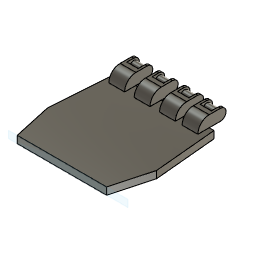
baseplate with holes (Autodesk Fusion 360 design; units mm, degrees)
Autodesk Fusion 360 part; units mm, degrees
sketch "Sketch1" plane through (0, 0, 0) normal (0, 0, 1) x (1, 0, 0)
  line L0 (0, 0) -> (76, 0)
  line L1 (76, 0) -> (76, 76)
  line L2 (76, 76) -> (0, 76)
  line L3 (0, 76) -> (0, 0)
  dimension "d1" = 76
  dimension "d2" = 76
  constraint horizontal L0
  constraint vertical L1
  constraint horizontal L2
  constraint vertical L3
  constraint coincident L0.start L3.end
  measures "d1" distance of L0.start L0.end
  measures "d2" distance of L0.start L2.end
extrude "Extrude1" add sketch "Sketch1" along normal blind 6.35
sketch "Sketch2" plane through (0, 0, 6.35) normal (0, 0, 1) x (-1, 0, 0)
  line L0 (0, -76) -> (0, 0)
  line L1 (0, 0) -> (-76, 0)
  line L2 (-76, 0) -> (-76, -76)
  line L3 (-76, -76) -> (0, -76)
  line L4 (-52, -66) -> (-38, -66)
  line L5 (-38, -66) -> (-38, -91)
  line L6 (-38, -91) -> (-52, -91)
  line L7 (-52, -91) -> (-52, -66)
  line L8 (-34.5, -66) -> (-20.5, -66)
  line L9 (-34.5, -91) -> (-34.5, -66)
  line L10 (-20.5, -66) -> (-20.5, -91)
  line L11 (-20.5, -91) -> (-34.5, -91)
  line L12 (-17, -66) -> (-3, -66)
  line L13 (-17, -91) -> (-17, -66)
  line L14 (-3, -66) -> (-3, -91)
  line L15 (-3, -91) -> (-17, -91)
  line L16 (-72, -66) -> (-58, -66)
  line L17 (-72, -91) -> (-72, -66)
  line L18 (-58, -66) -> (-58, -91)
  line L19 (-58, -91) -> (-72, -91)
  dimension "d5" = 14
  dimension "d6" = 25
  dimension "d7" = 24
  dimension "d8" = 10
  dimension "d89" = 35
  dimension "d90" = 0
  dimension "d93" = -20
  dimension "d94" = 0
  constraint horizontal L4
  constraint vertical L5
  constraint horizontal L6
  constraint vertical L7
  measures "d5" distance of L4.start L4.end
  measures "d6" distance of L4.start L6.end
  measures "d7" distance of L2 L7
  measures "d8" distance of L3 L4
extrude "Extrude2" add sketch "Sketch2" along normal blind 10 contours L3 L5 L6 L7 | L3 L4 L5 L7
fillet "Fillet1" radius 10 1 edges at (45, 66, 16.35)
fillet "Fillet2" radius 5 2 edges at (45, 91, 16.35) (45, 91, 6.35)
sketch "Sketch3" plane through (0, 0, 16.35) normal (0, 0, 1) x (-1, 0, 0)
  line L0 (-52, -86) -> (-38, -86)
  line L1 (-38, -86) -> (-38, -76)
  line L2 (-38, -76) -> (-52, -76)
  line L3 (-52, -76) -> (-52, -86)
  line L4 (-50, -80) -> (-40, -80)
  line L5 (-40, -80) -> (-40, -95)
  line L6 (-40, -95) -> (-50, -95)
  line L7 (-50, -95) -> (-50, -80)
  constraint horizontal L4
  constraint vertical L5
  constraint horizontal L6
  constraint vertical L7
extrude "Extrude3" cut sketch "Sketch3" against normal blind 20 contours L0 L4 L5 L7 | L0 L5 L6 L7
sketch "Sketch4" plane through (40, 0, 0) normal (1, 0, 0) x (0, 1, 0)
  line L0 (80, 6.35) -> (86, 6.35)
  arc A0 (86, 6.35) -> (86, 16.35) centre (86, 11.35) ccw
  line L1 (86, 16.35) -> (80, 16.35)
  line L2 (80, 16.35) -> (80, 6.35)
  circle A1 centre (86, 11.35) radius 3.25
  dimension "d17" = 6.5
  constraint concentric A0 A1
  measures "d17" diameter of A1
extrude "Extrude4" add sketch "Sketch4" along normal blind 10 contours A1
extrude "Extrude5" add 1 faces at (76, 25.3333, 2.1167) along direction (1, 0, 0) blind 5
extrude "Extrude6" add 1 faces at (0, 50.6667, 2.1167) along direction (-1, 0, 0) blind 5
extrude "Extrude7" add 1 faces at (23.6667, 0, 2.1167) along direction (0, -1, 0) blind 5
sketch "Sketch5" plane through (0, 0, 6.35) normal (0, 0, 1) x (-1, 0, 0)
  line L0 (-38, -66) -> (-38, -76)
  line L1 (-38, -76) -> (5, -76)
  line L2 (5, -76) -> (5, 5)
  line L3 (5, 5) -> (-81, 5)
  line L4 (-81, 5) -> (-81, -76)
  line L5 (-81, -76) -> (-52, -76)
  line L6 (-52, -76) -> (-52, -66)
  line L7 (-52, -66) -> (-38, -66)
  line L8 (-81, -76) -> (-76.6575, -76)
  line L9 (-76.6575, -76) -> (-76.6575, -71)
  line L10 (-76.6575, -71) -> (-81, -71)
  line L11 (-81, -71) -> (-81, -76)
  line L12 (5, -76) -> (0, -76)
  line L13 (0, -76) -> (0, -71)
  line L14 (0, -71) -> (5, -71)
  line L15 (5, -71) -> (5, -76)
  line L16 (5, 5) -> (0, 5)
  line L17 (0, 5) -> (0, 0)
  line L18 (0, 0) -> (5, 0)
  line L19 (5, 0) -> (5, 5)
  line L20 (-81, 5) -> (-76, 5)
  line L21 (-76, 5) -> (-76, 0)
  line L22 (-76, 0) -> (-81, 0)
  line L23 (-81, 0) -> (-81, 5)
  dimension "d26" = 5
  dimension "d27" = 5
  dimension "d28" = 5
  dimension "d29" = 5
  dimension "d30" = 5
  dimension "d31" = 5
  dimension "d32" = 5
  constraint horizontal L8
  constraint vertical L9
  constraint horizontal L10
  constraint vertical L11
  constraint coincident L4.end L5.start
  constraint horizontal L12
  constraint vertical L13
  constraint horizontal L14
  constraint vertical L15
  constraint coincident L1.end L2.start
  constraint horizontal L16
  constraint vertical L17
  constraint horizontal L18
  constraint vertical L19
  constraint coincident L2.end L3.start
  constraint horizontal L20
  constraint vertical L21
  constraint horizontal L22
  constraint vertical L23
  constraint coincident L3.end L4.start
  measures "d26" distance of L4.end L10.end
  measures "d27" distance of L1.end L12.end
  measures "d28" distance of L1.end L14.end
  measures "d29" distance of L2.end L16.end
  measures "d30" distance of L2.end L18.end
  measures "d31" distance of L3.end L20.end
  measures "d32" distance of L3.end L22.end
sketch "Sketch7" plane through (0, 0, 6.35) normal (0, 0, 1) x (-1, 0, 0)
  line L0 (5, 5) -> (-81, 5)
  line L1 (-81, 5) -> (-81, -76)
  line L2 (-38, -76) -> (5, -76)
  line L3 (-52, -76) -> (-52, -66)
  line L4 (-52, -66) -> (-38, -66)
  line L5 (-38, -66) -> (-38, -76)
  line L6 (5, -76) -> (5, 5)
  circle A0 centre (-38, -24.9192) radius 1
  circle A1 centre (-64, -24.9192) radius 1
  line L7 (-81, -76) -> (-52, -76)
  dimension "d35" = 2
  dimension "d36" = 2
  dimension "d39" = 26
  measures "d35" diameter of A1
  measures "d36" diameter of A0
  measures "d39" distance of A0.centre A1.centre
extrude "Extrude11" add 1 faces at (81, 22, 2.1167) along direction (1, 0, 0) blind 10
extrude "Extrude12" add 1 faces at (59, -5, 4.2333) along direction (0, -1, 0) blind 10
extrude "Extrude13" add 1 faces at (-5, 45.6667, 2.1167) along direction (-1, 0, 0) blind 10
sketch "Sketch10" plane through (0, -15, 0) normal (0, -1, 0) x (1, 0, 0)
  line L0 (-15, 0) -> (91, 0)
  line L1 (91, 0) -> (91, 6.35)
  line L2 (91, 6.35) -> (-15, 6.35)
  line L3 (-15, 6.35) -> (-15, 0)
sketch "Sketch11" plane through (0, 0, 0) normal (0, 0, 1) x (1, 0, 0)
  line L0 (91, 76) -> (96, 76)
  line L1 (96, 76) -> (96, 71)
  line L2 (96, 71) -> (91, 71)
  line L3 (91, 71) -> (91, 76)
  line L4 (-15, 76) -> (-20, 76)
  line L5 (-20, 76) -> (-20, 71)
  line L6 (-20, 71) -> (-15, 71)
  line L7 (-15, 71) -> (-15, 76)
  line L8 (91, -15) -> (86, -15)
  line L9 (86, -15) -> (86, -20)
  line L10 (86, -20) -> (91, -20)
  line L11 (91, -20) -> (91, -15)
  line L12 (-15, -15) -> (-10, -15)
  line L13 (-10, -15) -> (-10, -20)
  line L14 (-10, -20) -> (-15, -20)
  line L15 (-15, -20) -> (-15, -15)
  dimension "d70" = 5
  dimension "d71" = 5
  dimension "d72" = 5
  dimension "d73" = 5
  dimension "d74" = 5
  dimension "d75" = 5
  dimension "d76" = 5
  dimension "d77" = 5
  constraint horizontal L0
  constraint vertical L1
  constraint horizontal L2
  constraint vertical L3
  constraint horizontal L4
  constraint vertical L5
  constraint horizontal L6
  constraint vertical L7
  constraint horizontal L8
  constraint vertical L9
  constraint horizontal L10
  constraint vertical L11
  constraint horizontal L12
  constraint vertical L13
  constraint horizontal L14
  constraint vertical L15
  measures "d70" distance of L0.start L0.end
  measures "d71" distance of L0.start L2.end
  measures "d72" distance of L4.start L4.end
  measures "d73" distance of L4.start L6.end
  measures "d74" distance of L8.start L8.end
  measures "d75" distance of L8.start L10.end
  measures "d76" distance of L12.start L12.end
  measures "d77" distance of L12.start L14.end
sketch "Sketch12" plane through (0, 0, 0) normal (0, 0, 1) x (1, 0, 0)
  arc A0 (91, -20) -> (96, 71) centre (-640.4348, 65.8261) ccw
  arc A1 (-20, 71) -> (-15, -20) centre (801.5, 70.5) ccw
  arc A2 (-10, -20) -> (86, -20) centre (38, 315.1878) ccw
  line L0 (-20, 71) -> (-15, 71)
  line L1 (-15, 71) -> (-15, -20)
  line L2 (-10, -20) -> (-10, -14.8)
  line L3 (-10, -14.8) -> (86, -14)
  line L4 (86, -14) -> (86, -20)
  line L5 (96, 71) -> (90, 71)
  line L6 (90, 71) -> (90, -20)
  line L7 (90, -20) -> (91, -20)
  point P0 (-9.9984, -14.9986)
  constraint horizontal L0
  constraint vertical L2
  constraint parallel L2 L4
  constraint perpendicular L4 L5
  constraint perpendicular L5 L6
  constraint perpendicular L6 L7
pattern_linear "R-Pattern1" count 3 spacing 22.5 along (-1, 0, 0) of "Extrude2", "Fillet1", "Fillet2", "Extrude3", "Extrude4"
pattern_linear "R-Pattern2" count 2 spacing 20 along (1, 0, 0) of "Extrude2", "Fillet1", "Fillet2", "Extrude3", "Extrude4"
sketch "Sketch14" plane through (0, 0, 6.35) normal (0, 0, 1) x (-1, 0, 0)
  line L0 (-58, -66) -> (-58, -76)
  line L1 (-58, -76) -> (-52, -76)
  line L2 (-52, -76) -> (-52, -66)
  line L3 (-52, -66) -> (-38, -66)
  line L4 (-38, -66) -> (-38, -76)
  line L5 (-38, -76) -> (-29.5, -76)
  line L6 (-29.5, -76) -> (-29.5, -66)
  line L7 (-29.5, -66) -> (-15.5, -66)
  line L8 (-15.5, -66) -> (-15.5, -76)
  line L9 (-15.5, -76) -> (-7, -76)
  line L10 (-7, -76) -> (-7, -66)
  line L11 (-7, -66) -> (7, -66)
  line L12 (7, -66) -> (7, -76)
  line L13 (7, -76) -> (15, -76)
  line L14 (15, -76) -> (15, 15)
  line L15 (15, 15) -> (-91, 15)
  line L16 (-91, 15) -> (-91, -76)
  line L17 (-91, -76) -> (-72, -76)
  line L18 (-72, -76) -> (-72, -66)
  line L19 (-72, -66) -> (-58, -66)
  line L20 (-76.2804, -76) -> (-81.5, -19.824)
  line L21 (-81.5, -19.824) -> (-72, 15)
  line L22 (-72, 15) -> (7.2884, 15)
  line L23 (11, -76) -> (15, -19.824)
  line L24 (15, -19.824) -> (7.2884, 15)
  dimension "d105" = 56.176
  dimension "d106" = 56.176
  dimension "d107" = 102.486
  dimension "d108" = 105.259
  dimension "d109" = 87.2804
  dimension "d110" = 159.433
  constraint coincident L17 L20.start
  constraint coincident L15 L21.end
  constraint coincident L15 L22.end
  constraint midpoint L13 L23.start
  constraint coincident L14 L23.end
  measures "d105" vertical distance of L20.start L20.end
  measures "d106" vertical distance of L23.start L23.end
  measures "d107" angle of L22 L24
  measures "d108" angle of L21 L22
  measures "d109" distance of L20.start L23.start
  measures "d110" angle of L20 L21
extrude "Extrude17" cut sketch "Sketch14" against normal blind 10 contours L15 L16 L17 L20 L21 | L14 L15 L24 | L13 L14 L23
sketch "Sketch15" plane through (0, 0, 0) normal (0, 0, -1) x (1, 0, 0)
  line L0 (-15, -19.824) -> (-11, -76)
  line L1 (-11, -76) -> (76.2804, -76)
  line L2 (76.2804, -76) -> (81.5, -19.824)
  line L3 (81.5, -19.824) -> (72, 15)
  line L4 (72, 15) -> (-7.2884, 15)
  line L5 (-7.2884, 15) -> (-15, -19.824)
  line L6 (73.0232, -74) -> (57.0232, -74)
  line L7 (57.0232, -74) -> (57.0232, -25.5)
  line L8 (57.0232, -25.5) -> (73.0232, -25.5)
  line L9 (73.0232, -25.5) -> (73.0232, -74)
  line L10 (52.9695, -74) -> (36.9695, -74)
  line L11 (36.9695, -74) -> (36.9695, -25.5)
  line L12 (36.9695, -25.5) -> (52.9695, -25.5)
  line L13 (52.9695, -25.5) -> (52.9695, -74)
  line L14 (30.4888, -74) -> (14.4888, -74)
  line L15 (14.4888, -74) -> (14.4888, -25.5)
  line L16 (14.4888, -25.5) -> (30.4888, -25.5)
  line L17 (30.4888, -25.5) -> (30.4888, -74)
  line L18 (8.0069, -74) -> (-7.9931, -74)
  line L19 (-7.9931, -74) -> (-7.9931, -25.5)
  line L20 (-7.9931, -25.5) -> (8.0069, -25.5)
  line L21 (8.0069, -25.5) -> (8.0069, -74)
  dimension "d113" = 16
  dimension "d114" = 16
  dimension "d115" = 16
  dimension "d116" = 16
  dimension "d117" = 48.5
  dimension "d118" = 48.5
  dimension "d119" = 48.5
  dimension "d120" = 48.5
  dimension "d121" = 2
  dimension "d122" = 2
  dimension "d123" = 2
  dimension "d124" = 2
  dimension "d125" = 4.0537
  dimension "d126" = 90
  dimension "d127" = 6.4807
  dimension "d128" = 6.4819
  dimension "d129" = 3.2572
  constraint parallel L1 L6
  constraint perpendicular L6 L7
  constraint perpendicular L7 L8
  constraint perpendicular L6 L9
  constraint perpendicular L9 L10
  constraint perpendicular L10 L11
  constraint perpendicular L11 L12
  constraint perpendicular L10 L13
  constraint perpendicular L11 L14
  constraint perpendicular L14 L15
  constraint perpendicular L15 L16
  constraint perpendicular L15 L18
  constraint perpendicular L18 L19
  constraint perpendicular L19 L20
  constraint perpendicular L18 L21
  measures "d113" distance of L6.start L6.end
  measures "d114" distance of L10.start L10.end
  measures "d115" distance of L14.start L14.end
  measures "d116" distance of L18.start L18.end
  measures "d117" distance of L18.end L19.end
  measures "d118" distance of L14.end L15.end
  measures "d119" distance of L10.end L11.end
  measures "d120" distance of L6.start L8.end
  measures "d121" distance of L1 L6
  measures "d122" distance of L1 L10
  measures "d123" distance of L1 L18
  measures "d124" distance of L1 L14
  measures "d125" distance of L7 L13
  measures "d126" angle of L16 L17
  measures "d127" distance of L11 L17
  measures "d128" distance of L15 L21
  measures "d129" horizontal distance of L1.end L6.start
extrude "Extrude18" cut sketch "Sketch15" against normal blind 5 contours L6 L7 L8 L9 | L10 L11 L12 L13 | L14 L15 L16 L17 | L18 L19 L20 L21
sketch "Sketch16" plane through (0, 0, 0) normal (0, 0, -1) x (1, 0, 0)
  line L0 (36.9695, -74) -> (36.9695, -25.5)
  line L1 (36.9695, -25.5) -> (52.9695, -25.5)
  line L2 (52.9695, -25.5) -> (52.9695, -74)
  line L3 (52.9695, -74) -> (36.9695, -74)
  line L4 (14.4888, -74) -> (14.4888, -25.5)
  line L5 (14.4888, -25.5) -> (30.4888, -25.5)
  line L6 (30.4888, -25.5) -> (30.4888, -74)
  line L7 (30.4888, -74) -> (14.4888, -74)
  line L8 (57.0232, -74) -> (57.0232, -25.5)
  line L9 (57.0232, -25.5) -> (73.0232, -25.5)
  line L10 (73.0232, -25.5) -> (73.0232, -74)
  line L11 (73.0232, -74) -> (57.0232, -74)
  line L12 (-7.9931, -74) -> (-7.9931, -25.5)
  line L13 (-7.9931, -25.5) -> (8.0069, -25.5)
  line L14 (8.0069, -25.5) -> (8.0069, -74)
  line L15 (8.0069, -74) -> (-7.9931, -74)
  line L16 (-15, -19.824) -> (-11, -76)
  line L17 (-11, -76) -> (76.2804, -76)
  line L18 (76.2804, -76) -> (81.5, -19.824)
  line L19 (81.5, -19.824) -> (72, 15)
  line L20 (72, 15) -> (-7.2884, 15)
  line L21 (-7.2884, 15) -> (-15, -19.824)
  circle A0 centre (34, -73) radius 0.5
  circle A1 centre (77.5, -23.5) radius 0.5
  circle A2 centre (33.7295, -27.5) radius 0.5
  circle A3 centre (-11.9931, -22) radius 0.5
  dimension "d132" = 1
  dimension "d133" = 3.5112
  dimension "d134" = 3
  dimension "d135" = 1
  dimension "d136" = 4
  dimension "d137" = 2
  dimension "d138" = 1
  dimension "d139" = 3.24
  dimension "d140" = 2
  dimension "d141" = 1
  dimension "d142" = 3.5
  dimension "d143" = 4
  measures "d132" diameter of A0
  measures "d133" distance of L6 A0.centre
  measures "d134" distance of L17 A0.centre
  measures "d135" diameter of A1
  measures "d136" horizontal distance of L18.end A1.centre
  measures "d137" distance of L9 A1.centre
  measures "d138" diameter of A2
  measures "d139" distance of L0 A2.centre
  measures "d140" distance of L5 A2.centre
  measures "d141" diameter of A3
  measures "d142" distance of L13 A3.centre
  measures "d143" distance of L12 A3.centre
hole "Hole3" at (34, 73, 0) at (77.5, 23.5, 0) at (33.7295, 27.5, 0) at (-11.9931, 22, 0) direction (0, 0, 1) diameter 1 depth 2 tip angle 118
